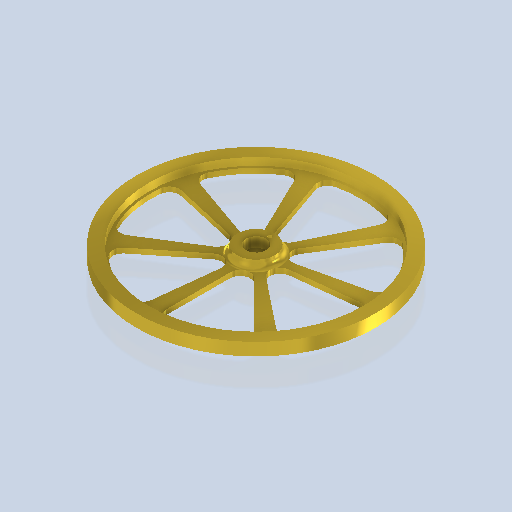
# Autodesk Inventor part: Wheel
Saved by Autodesk Inventor 2024.2 (Build 282272000, 272)
## iProperties
Created: 2024-04-02
Part Number: Wheel
Material: Gold
Document SubType Name: Modeling
Designer: ffogue
Density: 19.3 g/cm^3
Appearance: Metall - 2400F (heiß)
Author: ffogue
Autodesk Inventor part; units mm, degrees
ref_plane "YZ Plane" through (0, 0, 0) normal (1, 0, 0) x (0, 1, 0)
ref_plane "XZ Plane" through (0, 0, 0) normal (0, 1, 0) x (-1, 0, 0)
ref_plane "XY Plane" through (0, 0, 0) normal (0, 0, 1) x (1, 0, 0)
sketch "Skizze1" plane through (0, 0, 0) normal (0, 0, 1) x (1, 0, 0)
  circle A0 centre (0, 0) radius 47.5
  dimension "d0" = 95
  constraints: 1 centre point, 1 coincident
  measures "d0" diameter of A0
extrude "Extrusion1" add sketch "Skizze1" along normal blind 5
sketch "Skizze6" plane through (0, 0, 5) normal (0, 0, 1) x (1, 0, 0)
  circle A0 centre (0, 0) radius 42.5
  dimension "d18" = 85
  constraints: 1 centre point, 1 coincident
  measures "d18" diameter of A0
extrude "Extrusion4" cut sketch "Skizze6" against normal blind 3
sketch "Skizze8" plane through (0, 0, 2) normal (0, 0, 1) x (1, 0, 0)
  circle A0 centre (0, 0) radius 7.5
  dimension "d24" = 15
  constraints: 1 centre point, 1 coincident
  measures "d24" diameter of A0
extrude "Extrusion6" add sketch "Skizze8" along normal up to surface (3 mm away)
sketch "Skizze9" plane through (0, 0, 5) normal (0, 0, 1) x (1, 0, 0)
  circle A0 centre (0, 0) radius 7.5 projected
  constraints: 1 coincident
hole "Bohrung2" at (0, 0, 5) direction (0, 0, -1) diameter 3 end through all counterbore diameter 8 counterbore depth 4
sketch "Skizze10" plane through (0, 0, 0) normal (0, 0, -1) x (-1, 0, 0)
  circle A0 centre (0, 0) radius 1.5 projected
  circle A1 centre (0, 0) radius 2.5
  dimension "d34" = 5
  constraints: 1 centre point, 1 coincident
  measures "d34" diameter of A1
extrude "Extrusion7" add sketch "Skizze10" along normal blind 3
sketch "Skizze11" plane through (0, 0, 2) normal (0, 0, 1) x (1, 0, 0)
  circle A0 centre (0, 0) radius 1.5 projected
  circle A1 centre (0, 0) radius 41.5 construction
  circle A2 centre (0, 0) radius 4 projected
  line L0 (0, 0) -> (0, -51.5303) construction
  circle A3 centre (0, 0) radius 7.5 projected
  circle A4 centre (0, 0) radius 8.676 construction
  line L1 (1.5, -11.8019) -> (1.5, -37.0945)
  arc A5 (1.5, -37.0945) -> (6.0867, -41.0512) centre (5.5, -37.0945) ccw
  arc A6 (6.0867, -41.0512) -> (25.65, -32.6241) centre (0, 0) ccw
  arc A7 (25.65, -32.6241) -> (26.0061, -26.6512) centre (23.1777, -29.4796) ccw
  line L2 (26.0061, -26.6512) -> (8.3284, -8.9735)
  arc A8 (8.3284, -8.9735) -> (1.5, -11.8019) centre (5.5, -11.8019) ccw
  line L3 (0, 0) -> (38.2001, -38.2001) construction
  dimension "d37" = 83
  dimension "d38" = 17.352
  dimension "d39" = 1.5
  dimension "d40" = 45
  dimension "d41" = 4
  dimension "d42" = 41.5
  dimension "d43" = 25
  dimension "d44" = 4
  constraints: 8 end point, 8 point on circle, 6 centre point, 6 tangent, 2 coincident, 2 vertical, 1 concentric, 1 equal radius, 1 parallel
  measures "d37" diameter of A1
  measures "d38" diameter of A4
  measures "d39" distance between parallel lines of L0 L1
  measures "d40" angle of L3 L0
  measures "d41" radius of A7
  measures "d42" radius of A6
  measures "d43" distance of A8.centre A7.centre
  measures "d44" radius of A8
extrude "Extrusion8" cut sketch "Skizze11" against normal up to surface (2 mm away) contours A8 L2 A7 A6 A5 L1
pattern_circular "Runde Anordnung1" count 7 over 360 about axis through (0, 0, 5) along (0, 0, -1) of "Extrusion8"
fillet "Rundung1" radius 2 1 edges at (-7.5, 0, 2)
sketch "Skizze12" plane through (0, 0, 0) normal (0, 0, -1) x (-1, 0, 0)
  point P0 (0, 0)
  point P1 (0.0019, 5.5)
  dimension "d58" = 5.5
  measures "d58" distance of point (0.002, 5.5) point (0, 0)
hole "Bohrung3" at (-0.0019, 5.5, 0) direction (0, 0, 1) diameter 1.6 end through all
